Autodesk Inventor part; units mm, degrees
(part 2 of 2)
  spline S369 degree 3 poles (263.9908, 122.8577) (263.1328, 122.8577) (262.3593, 122.3409) (262.031, 121.5482) knots 0 0 0 0 1 1 1 1 projected
  spline S370 degree 3 poles (262.4908, 119.2364) (263.0975, 118.6297) (264.0099, 118.4482) (264.8026, 118.7766) knots 0 0 0 0 1 1 1 1 projected
  spline S371 degree 3 poles (265.4908, 122.2364) (265.093, 122.6342) (264.5534, 122.8577) (263.9908, 122.8577) knots 0 0 0 0 1 1 1 1 projected
  spline S372 degree 3 poles (266.1121, 120.7364) (266.1121, 121.299) (265.8886, 121.8386) (265.4908, 122.2364) knots 0 0 0 0 1 1 1 1 projected
  spline S373 degree 3 poles (264.8026, 118.7766) (265.5953, 119.1049) (266.1121, 119.8784) (266.1121, 120.7364) knots 0 0 0 0 1 1 1 1 projected
  spline S374 degree 3 poles (252.3068, 94.2009) (251.4488, 94.2009) (250.6753, 93.6841) (250.347, 92.8914) knots 0 0 0 0 1 1 1 1 projected
  spline S375 degree 3 poles (250.347, 92.8914) (250.0186, 92.0987) (250.2001, 91.1863) (250.8068, 90.5796) knots 0 0 0 0 1 1 1 1 projected
  spline S376 degree 3 poles (253.8068, 93.5796) (253.409, 93.9774) (252.8694, 94.2009) (252.3068, 94.2009) knots 0 0 0 0 1 1 1 1 projected
  spline S377 degree 3 poles (254.4281, 92.0796) (254.4281, 92.6422) (254.2046, 93.1818) (253.8068, 93.5796) knots 0 0 0 0 1 1 1 1 projected
  spline S378 degree 3 poles (253.1186, 90.1198) (253.9113, 90.4481) (254.4281, 91.2216) (254.4281, 92.0796) knots 0 0 0 0 1 1 1 1 projected
  spline S379 degree 3 poles (250.8068, 90.5796) (251.4135, 89.9729) (252.3259, 89.7914) (253.1186, 90.1198) knots 0 0 0 0 1 1 1 1 projected
  spline S380 degree 3 poles (249.25, 11.25) (249.25, 11.7141) (249.0656, 12.1592) (248.7374, 12.4874) knots 0 0 0 0 1 1 1 1 projected
  spline S381 degree 3 poles (248.1697, 9.6332) (248.8236, 9.9041) (249.25, 10.5422) (249.25, 11.25) knots 0 0 0 0 1 1 1 1 projected
  spline S382 degree 3 poles (257.9446, 32.9698) (258.7373, 33.2981) (259.2541, 34.0716) (259.2541, 34.9296) knots 0 0 0 0 1 1 1 1 projected
  spline S383 degree 3 poles (248.7374, 12.4874) (248.4092, 12.8156) (247.9641, 13) (247.5, 13) knots 0 0 0 0 1 1 1 1 projected
  spline S384 degree 3 poles (246.2626, 10.0126) (246.7631, 9.5121) (247.5158, 9.3623) (248.1697, 9.6332) knots 0 0 0 0 1 1 1 1 projected
  spline S385 degree 3 poles (247.5, 13) (246.7922, 13) (246.1541, 12.5736) (245.8832, 11.9197) knots 0 0 0 0 1 1 1 1 projected
  spline S386 degree 3 poles (245.8832, 107.0581) (245.6123, 106.4042) (245.7621, 105.6515) (246.2626, 105.151) knots 0 0 0 0 1 1 1 1 projected
  spline S387 degree 3 poles (245.8832, 11.9197) (245.6123, 11.2658) (245.7621, 10.5131) (246.2626, 10.0126) knots 0 0 0 0 1 1 1 1 projected
  spline S388 degree 3 poles (255.173, 35.7414) (254.8446, 34.9487) (255.0261, 34.0363) (255.6328, 33.4296) knots 0 0 0 0 1 1 1 1 projected
  line L32 (240.6245, 24.8046) -> (240.6245, 9.8046) projected
  spline S389 degree 3 poles (259.2541, 34.9296) (259.2541, 35.4922) (259.0306, 36.0318) (258.6328, 36.4296) knots 0 0 0 0 1 1 1 1 projected
  line L33 (234.6245, 24.8046) -> (240.6245, 24.8046) projected
  spline S390 degree 3 poles (239.5768, 36.4076) (239.179, 36.8054) (238.6394, 37.0289) (238.0768, 37.0289) knots 0 0 0 0 1 1 1 1 projected
  spline S391 degree 3 poles (240.1981, 34.9076) (240.1981, 35.4702) (239.9746, 36.0098) (239.5768, 36.4076) knots 0 0 0 0 1 1 1 1 projected
  spline S392 degree 3 poles (238.8886, 32.9478) (239.6813, 33.2761) (240.1981, 34.0496) (240.1981, 34.9076) knots 0 0 0 0 1 1 1 1 projected
  spline S393 degree 3 poles (236.5768, 33.4076) (237.1835, 32.8009) (238.0959, 32.6194) (238.8886, 32.9478) knots 0 0 0 0 1 1 1 1 projected
  spline S394 degree 3 poles (236.117, 35.7194) (235.7886, 34.9267) (235.9701, 34.0143) (236.5768, 33.4076) knots 0 0 0 0 1 1 1 1 projected
  spline S395 degree 3 poles (238.0768, 37.0289) (237.2188, 37.0289) (236.4453, 36.5121) (236.117, 35.7194) knots 0 0 0 0 1 1 1 1 projected
  spline S396 degree 3 poles (249.8561, 53.9796) (249.8561, 54.5422) (249.6326, 55.0818) (249.2348, 55.4796) knots 0 0 0 0 1 1 1 1 projected
  spline S397 degree 3 poles (248.5466, 52.0198) (249.3393, 52.3481) (249.8561, 53.1216) (249.8561, 53.9796) knots 0 0 0 0 1 1 1 1 projected
  spline S398 degree 3 poles (249.2348, 55.4796) (248.837, 55.8774) (248.2974, 56.1009) (247.7348, 56.1009) knots 0 0 0 0 1 1 1 1 projected
  spline S399 degree 3 poles (246.2348, 52.4796) (246.8415, 51.8729) (247.7539, 51.6914) (248.5466, 52.0198) knots 0 0 0 0 1 1 1 1 projected
  spline S400 degree 3 poles (247.7348, 56.1009) (246.8768, 56.1009) (246.1033, 55.5841) (245.775, 54.7914) knots 0 0 0 0 1 1 1 1 projected
  spline S401 degree 3 poles (230.5521, 53.9796) (230.5521, 54.5422) (230.3286, 55.0818) (229.9308, 55.4796) knots 0 0 0 0 1 1 1 1 projected
  spline S402 degree 3 poles (229.2426, 52.0198) (230.0353, 52.3481) (230.5521, 53.1216) (230.5521, 53.9796) knots 0 0 0 0 1 1 1 1 projected
  spline S403 degree 3 poles (229.9308, 55.4796) (229.533, 55.8774) (228.9934, 56.1009) (228.4308, 56.1009) knots 0 0 0 0 1 1 1 1 projected
  spline S404 degree 3 poles (245.775, 54.7914) (245.4466, 53.9987) (245.6281, 53.0863) (246.2348, 52.4796) knots 0 0 0 0 1 1 1 1 projected
  spline S405 degree 3 poles (225.1048, 74.5296) (224.707, 74.9274) (224.1674, 75.1509) (223.6048, 75.1509) knots 0 0 0 0 1 1 1 1 projected
  spline S406 degree 3 poles (223.6048, 75.1509) (222.7468, 75.1509) (221.9733, 74.6341) (221.645, 73.8414) knots 0 0 0 0 1 1 1 1 projected
  spline S407 degree 3 poles (225.7261, 73.0296) (225.7261, 73.5922) (225.5026, 74.1318) (225.1048, 74.5296) knots 0 0 0 0 1 1 1 1 projected
  spline S408 degree 3 poles (221.645, 73.8414) (221.3166, 73.0487) (221.4981, 72.1363) (222.1048, 71.5296) knots 0 0 0 0 1 1 1 1 projected
  spline S409 degree 3 poles (222.1048, 71.5296) (222.7115, 70.9229) (223.6239, 70.7414) (224.4166, 71.0698) knots 0 0 0 0 1 1 1 1 projected
  spline S410 degree 3 poles (224.4166, 71.0698) (225.2093, 71.3981) (225.7261, 72.1716) (225.7261, 73.0296) knots 0 0 0 0 1 1 1 1 projected
  spline S411 degree 3 poles (244.1548, 74.5296) (243.757, 74.9274) (243.2174, 75.1509) (242.6548, 75.1509) knots 0 0 0 0 1 1 1 1 projected
  spline S412 degree 3 poles (240.695, 73.8414) (240.3666, 73.0487) (240.5481, 72.1363) (241.1548, 71.5296) knots 0 0 0 0 1 1 1 1 projected
  spline S413 degree 3 poles (244.7761, 73.0296) (244.7761, 73.5922) (244.5526, 74.1318) (244.1548, 74.5296) knots 0 0 0 0 1 1 1 1 projected
  spline S414 degree 3 poles (241.1548, 71.5296) (241.7615, 70.9229) (242.6739, 70.7414) (243.4666, 71.0698) knots 0 0 0 0 1 1 1 1 projected
  spline S415 degree 3 poles (243.4666, 71.0698) (244.2593, 71.3981) (244.7761, 72.1716) (244.7761, 73.0296) knots 0 0 0 0 1 1 1 1 projected
  spline S416 degree 3 poles (242.6548, 75.1509) (241.7968, 75.1509) (241.0233, 74.6341) (240.695, 73.8414) knots 0 0 0 0 1 1 1 1 projected
  spline S417 degree 3 poles (241.6148, 122.2364) (241.217, 122.6342) (240.6774, 122.8577) (240.1148, 122.8577) knots 0 0 0 0 1 1 1 1 projected
  spline S418 degree 3 poles (242.2361, 120.7364) (242.2361, 121.299) (242.0126, 121.8386) (241.6148, 122.2364) knots 0 0 0 0 1 1 1 1 projected
  spline S419 degree 3 poles (240.9266, 118.7766) (241.7193, 119.1049) (242.2361, 119.8784) (242.2361, 120.7364) knots 0 0 0 0 1 1 1 1 projected
  spline S420 degree 3 poles (238.6148, 119.2364) (239.2215, 118.6297) (240.1339, 118.4482) (240.9266, 118.7766) knots 0 0 0 0 1 1 1 1 projected
  spline S421 degree 3 poles (240.1148, 122.8577) (239.2568, 122.8577) (238.4833, 122.3409) (238.155, 121.5482) knots 0 0 0 0 1 1 1 1 projected
  spline S422 degree 3 poles (238.155, 121.5482) (237.8266, 120.7555) (238.0081, 119.8431) (238.6148, 119.2364) knots 0 0 0 0 1 1 1 1 projected
  spline S423 degree 3 poles (235.3781, 92.0796) (235.3781, 92.6422) (235.1546, 93.1818) (234.7568, 93.5796) knots 0 0 0 0 1 1 1 1 projected
  spline S424 degree 3 poles (234.0686, 90.1198) (234.8613, 90.4481) (235.3781, 91.2216) (235.3781, 92.0796) knots 0 0 0 0 1 1 1 1 projected
  spline S425 degree 3 poles (234.7568, 93.5796) (234.359, 93.9774) (233.8194, 94.2009) (233.2568, 94.2009) knots 0 0 0 0 1 1 1 1 projected
  spline S426 degree 3 poles (231.7568, 90.5796) (232.3635, 89.9729) (233.2759, 89.7914) (234.0686, 90.1198) knots 0 0 0 0 1 1 1 1 projected
  spline S427 degree 3 poles (233.2568, 94.2009) (232.3988, 94.2009) (231.6253, 93.6841) (231.297, 92.8914) knots 0 0 0 0 1 1 1 1 projected
  spline S428 degree 3 poles (231.297, 92.8914) (230.9686, 92.0987) (231.1501, 91.1863) (231.7568, 90.5796) knots 0 0 0 0 1 1 1 1 projected
  spline S429 degree 3 poles (216.3281, 92.0796) (216.3281, 92.6422) (216.1046, 93.1818) (215.7068, 93.5796) knots 0 0 0 0 1 1 1 1 projected
  spline S430 degree 3 poles (215.0186, 90.1198) (215.8113, 90.4481) (216.3281, 91.2216) (216.3281, 92.0796) knots 0 0 0 0 1 1 1 1 projected
  spline S431 degree 3 poles (215.7068, 93.5796) (215.309, 93.9774) (214.7694, 94.2009) (214.2068, 94.2009) knots 0 0 0 0 1 1 1 1 projected
  spline S432 degree 3 poles (212.7068, 90.5796) (213.3135, 89.9729) (214.2259, 89.7914) (215.0186, 90.1198) knots 0 0 0 0 1 1 1 1 projected
  spline S433 degree 3 poles (212.247, 92.8914) (211.9186, 92.0987) (212.1001, 91.1863) (212.7068, 90.5796) knots 0 0 0 0 1 1 1 1 projected
  spline S434 degree 3 poles (214.2068, 94.2009) (213.3488, 94.2009) (212.5753, 93.6841) (212.247, 92.8914) knots 0 0 0 0 1 1 1 1 projected
  spline S435 degree 3 poles (217.0506, 118.7766) (217.8433, 119.1049) (218.3601, 119.8784) (218.3601, 120.7364) knots 0 0 0 0 1 1 1 1 projected
  spline S436 degree 3 poles (218.3601, 120.7364) (218.3601, 121.299) (218.1366, 121.8386) (217.7388, 122.2364) knots 0 0 0 0 1 1 1 1 projected
  spline S437 degree 3 poles (214.7388, 119.2364) (215.3455, 118.6297) (216.2579, 118.4482) (217.0506, 118.7766) knots 0 0 0 0 1 1 1 1 projected
  spline S438 degree 3 poles (217.7388, 122.2364) (217.341, 122.6342) (216.8014, 122.8577) (216.2388, 122.8577) knots 0 0 0 0 1 1 1 1 projected
  spline S439 degree 3 poles (216.2388, 122.8577) (215.3808, 122.8577) (214.6073, 122.3409) (214.279, 121.5482) knots 0 0 0 0 1 1 1 1 projected
  spline S440 degree 3 poles (214.279, 121.5482) (213.9506, 120.7555) (214.1321, 119.8431) (214.7388, 119.2364) knots 0 0 0 0 1 1 1 1 projected
  spline S441 degree 3 poles (221.1581, 34.9276) (221.1581, 36.0992) (220.2084, 37.0489) (219.0368, 37.0489) knots 0 0 0 0 1 1 1 1 projected
  spline S442 degree 3 poles (219.8486, 32.9678) (220.6413, 33.2961) (221.1581, 34.0696) (221.1581, 34.9276) knots 0 0 0 0 1 1 1 1 projected
  spline S443 degree 3 poles (217.5368, 33.4276) (218.1435, 32.8209) (219.0559, 32.6394) (219.8486, 32.9678) knots 0 0 0 0 1 1 1 1 projected
  spline S444 degree 3 poles (217.077, 35.7394) (216.7486, 34.9467) (216.9301, 34.0343) (217.5368, 33.4276) knots 0 0 0 0 1 1 1 1 projected
  spline S445 degree 3 poles (219.0368, 37.0489) (218.1788, 37.0489) (217.4053, 36.5321) (217.077, 35.7394) knots 0 0 0 0 1 1 1 1 projected
  spline S446 degree 3 poles (228.4308, 56.1009) (227.5728, 56.1009) (226.7993, 55.5841) (226.471, 54.7914) knots 0 0 0 0 1 1 1 1 projected
  spline S447 degree 3 poles (226.471, 54.7914) (226.1426, 53.9987) (226.3241, 53.0863) (226.9308, 52.4796) knots 0 0 0 0 1 1 1 1 projected
  spline S448 degree 3 poles (226.9308, 52.4796) (227.5375, 51.8729) (228.4499, 51.6914) (229.2426, 52.0198) knots 0 0 0 0 1 1 1 1 projected
  spline S449 degree 3 poles (211.5021, 53.9796) (211.5021, 54.5422) (211.2786, 55.0818) (210.8808, 55.4796) knots 0 0 0 0 1 1 1 1 projected
  spline S450 degree 3 poles (210.1926, 52.0198) (210.9853, 52.3481) (211.5021, 53.1216) (211.5021, 53.9796) knots 0 0 0 0 1 1 1 1 projected
  spline S451 degree 3 poles (209.3808, 56.1009) (208.5228, 56.1009) (207.7493, 55.5841) (207.421, 54.7914) knots 0 0 0 0 1 1 1 1 projected
  spline S452 degree 3 poles (207.8808, 52.4796) (208.4875, 51.8729) (209.3999, 51.6914) (210.1926, 52.0198) knots 0 0 0 0 1 1 1 1 projected
  spline S453 degree 3 poles (207.421, 54.7914) (207.0926, 53.9987) (207.2741, 53.0863) (207.8808, 52.4796) knots 0 0 0 0 1 1 1 1 projected
  spline S454 degree 3 poles (210.8808, 55.4796) (210.483, 55.8774) (209.9434, 56.1009) (209.3808, 56.1009) knots 0 0 0 0 1 1 1 1 projected
  line L34 (298.1708, 72.3776) -> (298.1708, 78.3776) projected
  line L35 (298.1708, 78.3776) -> (313.1708, 78.3776) projected
  line L36 (313.1708, 78.3776) -> (313.1708, 72.3776) projected
  line L37 (298.1708, 54.3776) -> (313.1708, 54.3776) projected
  line L38 (298.1708, 48.3776) -> (298.1708, 54.3776) projected
  line L39 (313.1708, 48.3776) -> (298.1708, 48.3776) projected
  line L40 (313.1708, 54.3776) -> (313.1708, 48.3776) projected
  line L41 (301.9468, 43.9296) -> (307.9468, 43.9296) projected
  spline S455 degree 3 poles (292.9468, 37.0509) (292.0888, 37.0509) (291.3153, 36.5341) (290.987, 35.7414) knots 0 0 0 0 1 1 1 1 projected
  spline S456 degree 3 poles (293.7586, 32.9698) (294.5513, 33.2981) (295.0681, 34.0716) (295.0681, 34.9296) knots 0 0 0 0 1 1 1 1 projected
  line L42 (277.9468, 43.9296) -> (283.9468, 43.9296) projected
  spline S457 degree 3 poles (291.4468, 33.4296) (292.0535, 32.8229) (292.9659, 32.6414) (293.7586, 32.9698) knots 0 0 0 0 1 1 1 1 projected
  line L43 (301.9468, 28.9296) -> (301.9468, 43.9296) projected
  line L44 (307.9468, 28.9296) -> (301.9468, 28.9296) projected
  line L45 (307.9468, 43.9296) -> (307.9468, 28.9296) projected
  line L46 (277.9468, 28.9296) -> (277.9468, 43.9296) projected
  line L47 (283.9468, 28.9296) -> (277.9468, 28.9296) projected
  spline S458 degree 3 poles (258.6328, 36.4296) (258.235, 36.8274) (257.6954, 37.0509) (257.1328, 37.0509) knots 0 0 0 0 1 1 1 1 projected
  spline S459 degree 3 poles (257.1328, 37.0509) (256.2748, 37.0509) (255.5013, 36.5341) (255.173, 35.7414) knots 0 0 0 0 1 1 1 1 projected
  spline S460 degree 3 poles (248.1697, 104.7716) (248.8236, 105.0425) (249.25, 105.6806) (249.25, 106.3884) knots 0 0 0 0 1 1 1 1 projected
  spline S461 degree 3 poles (249.25, 106.3884) (249.25, 106.8525) (249.0656, 107.2976) (248.7374, 107.6258) knots 0 0 0 0 1 1 1 1 projected
  spline S462 degree 3 poles (246.2626, 105.151) (246.7631, 104.6505) (247.5158, 104.5007) (248.1697, 104.7716) knots 0 0 0 0 1 1 1 1 projected
  spline S463 degree 3 poles (266.603, 16.6914) (266.2746, 15.8987) (266.4561, 14.9863) (267.0628, 14.3796) knots 0 0 0 0 1 1 1 1 projected
  spline S464 degree 3 poles (248.7374, 107.6258) (248.4092, 107.954) (247.9641, 108.1384) (247.5, 108.1384) knots 0 0 0 0 1 1 1 1 projected
  spline S465 degree 3 poles (247.5, 108.1384) (246.7922, 108.1384) (246.1541, 107.712) (245.8832, 107.0581) knots 0 0 0 0 1 1 1 1 projected
  line L48 (240.6245, 9.8046) -> (234.6245, 9.8046) projected
  line L49 (234.6245, 9.8046) -> (234.6245, 24.8046) projected
  line L50 (467.2088, 40.476) -> (452.2088, 40.476) projected
  line L51 (467.2088, 34.476) -> (467.2088, 40.476) projected
  line L52 (452.2088, 34.476) -> (467.2088, 34.476) projected
  line L53 (22.5, 6.25) -> (472.5, 6.25) projected
  line L54 (22.5, 131.25) -> (472.5, 131.25) projected
  line L55 (22.5, 131.25) -> (22.5, 6.25) projected
  spline S466 degree 3 poles (25.8832, 44.9197) (25.6123, 44.2658) (25.7621, 43.5131) (26.2626, 43.0126) knots 0 0 0 0 1 1 1 1 projected
  spline S467 degree 3 poles (27.5, 46) (26.7922, 46) (26.1541, 45.5736) (25.8832, 44.9197) knots 0 0 0 0 1 1 1 1 projected
  spline S468 degree 3 poles (319.4023, 126.7719) (318.4647, 127.7096) (317.1929, 128.2364) (315.8668, 128.2364) knots 0 0 0 0 1 1 1 1 projected
  spline S469 degree 3 poles (320.8668, 123.2364) (320.8668, 124.5625) (320.34, 125.8343) (319.4023, 126.7719) knots 0 0 0 0 1 1 1 1 projected
  spline S470 degree 3 poles (317.7802, 118.617) (319.6486, 119.3909) (320.8668, 121.2141) (320.8668, 123.2364) knots 0 0 0 0 1 1 1 1 projected
  spline S471 degree 3 poles (312.3313, 119.7009) (313.7613, 118.2709) (315.9118, 117.8431) (317.7802, 118.617) knots 0 0 0 0 1 1 1 1 projected
  spline S472 degree 3 poles (311.2474, 125.1498) (310.4735, 123.2814) (310.9013, 121.1309) (312.3313, 119.7009) knots 0 0 0 0 1 1 1 1 projected
  spline S473 degree 3 poles (315.8668, 128.2364) (313.8445, 128.2364) (312.0213, 127.0182) (311.2474, 125.1498) knots 0 0 0 0 1 1 1 1 projected
  spline S474 degree 3 poles (310.9568, 93.5796) (310.559, 93.9774) (310.0194, 94.2009) (309.4568, 94.2009) knots 0 0 0 0 1 1 1 1 projected
  spline S475 degree 3 poles (311.5781, 92.0796) (311.5781, 92.6422) (311.3546, 93.1818) (310.9568, 93.5796) knots 0 0 0 0 1 1 1 1 projected
  spline S476 degree 3 poles (309.4568, 89.9583) (310.6284, 89.9583) (311.5781, 90.908) (311.5781, 92.0796) knots 0 0 0 0 1 1 1 1 projected
  spline S477 degree 3 poles (307.3355, 92.0796) (307.3355, 90.908) (308.2852, 89.9583) (309.4568, 89.9583) knots 0 0 0 0 1 1 1 1 projected
  spline S478 degree 3 poles (309.4568, 94.2009) (308.2852, 94.2009) (307.3355, 93.2512) (307.3355, 92.0796) knots 0 0 0 0 1 1 1 1 projected
  spline S479 degree 3 poles (289.3668, 122.2364) (288.969, 122.6342) (288.4294, 122.8577) (287.8668, 122.8577) knots 0 0 0 0 1 1 1 1 projected
  spline S480 degree 3 poles (289.9881, 120.7364) (289.9881, 121.299) (289.7646, 121.8386) (289.3668, 122.2364) knots 0 0 0 0 1 1 1 1 projected
  spline S481 degree 3 poles (287.8668, 118.6151) (289.0384, 118.6151) (289.9881, 119.5648) (289.9881, 120.7364) knots 0 0 0 0 1 1 1 1 projected
  spline S482 degree 3 poles (285.7455, 120.7364) (285.7455, 119.5648) (286.6952, 118.6151) (287.8668, 118.6151) knots 0 0 0 0 1 1 1 1 projected
  spline S483 degree 3 poles (287.8668, 122.8577) (286.6952, 122.8577) (285.7455, 121.908) (285.7455, 120.7364) knots 0 0 0 0 1 1 1 1 projected
  spline S484 degree 3 poles (272.8568, 93.5796) (272.459, 93.9774) (271.9194, 94.2009) (271.3568, 94.2009) knots 0 0 0 0 1 1 1 1 projected
  spline S485 degree 3 poles (273.4781, 92.0796) (273.4781, 92.6422) (273.2546, 93.1818) (272.8568, 93.5796) knots 0 0 0 0 1 1 1 1 projected
  spline S486 degree 3 poles (272.1686, 90.1198) (272.9613, 90.4481) (273.4781, 91.2216) (273.4781, 92.0796) knots 0 0 0 0 1 1 1 1 projected
  spline S487 degree 3 poles (269.8568, 90.5796) (270.4635, 89.9729) (271.3759, 89.7914) (272.1686, 90.1198) knots 0 0 0 0 1 1 1 1 projected
  spline S488 degree 3 poles (269.397, 92.8914) (269.0686, 92.0987) (269.2501, 91.1863) (269.8568, 90.5796) knots 0 0 0 0 1 1 1 1 projected
  spline S489 degree 3 poles (271.3568, 94.2009) (270.4988, 94.2009) (269.7253, 93.6841) (269.397, 92.8914) knots 0 0 0 0 1 1 1 1 projected
  spline S490 degree 3 poles (288.447, 92.8914) (288.1186, 92.0987) (288.3001, 91.1863) (288.9068, 90.5796) knots 0 0 0 0 1 1 1 1 projected
  spline S491 degree 3 poles (290.4068, 94.2009) (289.5488, 94.2009) (288.7753, 93.6841) (288.447, 92.8914) knots 0 0 0 0 1 1 1 1 projected
  spline S492 degree 3 poles (288.9068, 90.5796) (289.5135, 89.9729) (290.4259, 89.7914) (291.2186, 90.1198) knots 0 0 0 0 1 1 1 1 projected
  spline S493 degree 3 poles (292.5281, 92.0796) (292.5281, 92.6422) (292.3046, 93.1818) (291.9068, 93.5796) knots 0 0 0 0 1 1 1 1 projected
  spline S494 degree 3 poles (291.2186, 90.1198) (292.0113, 90.4481) (292.5281, 91.2216) (292.5281, 92.0796) knots 0 0 0 0 1 1 1 1 projected
  spline S495 degree 3 poles (291.9068, 93.5796) (291.509, 93.9774) (290.9694, 94.2009) (290.4068, 94.2009) knots 0 0 0 0 1 1 1 1 projected
  spline S496 degree 3 poles (357.88, 36.4804) (357.4822, 36.8782) (356.9426, 37.1017) (356.38, 37.1017) knots 0 0 0 0 1 1 1 1 projected
  spline S497 degree 3 poles (358.5013, 34.9804) (358.5013, 35.543) (358.2778, 36.0826) (357.88, 36.4804) knots 0 0 0 0 1 1 1 1 projected
  spline S498 degree 3 poles (357.1918, 33.0206) (357.9845, 33.3489) (358.5013, 34.1224) (358.5013, 34.9804) knots 0 0 0 0 1 1 1 1 projected
  spline S499 degree 3 poles (354.88, 33.4804) (355.4867, 32.8737) (356.3991, 32.6922) (357.1918, 33.0206) knots 0 0 0 0 1 1 1 1 projected
  spline S500 degree 3 poles (356.38, 37.1017) (355.522, 37.1017) (354.7485, 36.5849) (354.4202, 35.7922) knots 0 0 0 0 1 1 1 1 projected
  spline S501 degree 3 poles (354.88, 52.5304) (355.4867, 51.9237) (356.3991, 51.7422) (357.1918, 52.0706) knots 0 0 0 0 1 1 1 1 projected
  spline S502 degree 3 poles (354.4202, 54.8422) (354.0918, 54.0495) (354.2733, 53.1371) (354.88, 52.5304) knots 0 0 0 0 1 1 1 1 projected
  spline S503 degree 3 poles (356.38, 56.1517) (355.522, 56.1517) (354.7485, 55.6349) (354.4202, 54.8422) knots 0 0 0 0 1 1 1 1 projected
  spline S504 degree 3 poles (357.88, 55.5304) (357.4822, 55.9282) (356.9426, 56.1517) (356.38, 56.1517) knots 0 0 0 0 1 1 1 1 projected
  spline S505 degree 3 poles (358.5013, 54.0304) (358.5013, 54.593) (358.2778, 55.1326) (357.88, 55.5304) knots 0 0 0 0 1 1 1 1 projected
  spline S506 degree 3 poles (357.1918, 52.0706) (357.9845, 52.3989) (358.5013, 53.1724) (358.5013, 54.0304) knots 0 0 0 0 1 1 1 1 projected
  spline S507 degree 3 poles (354.4202, 35.7922) (354.0918, 34.9995) (354.2733, 34.0871) (354.88, 33.4804) knots 0 0 0 0 1 1 1 1 projected
  spline S508 degree 3 poles (343.558, 93.6444) (343.1602, 94.0422) (342.6206, 94.2657) (342.058, 94.2657) knots 0 0 0 0 1 1 1 1 projected
  spline S509 degree 3 poles (344.1793, 92.1444) (344.1793, 92.707) (343.9558, 93.2466) (343.558, 93.6444) knots 0 0 0 0 1 1 1 1 projected
  spline S510 degree 3 poles (342.8698, 90.1846) (343.6625, 90.5129) (344.1793, 91.2864) (344.1793, 92.1444) knots 0 0 0 0 1 1 1 1 projected
  spline S511 degree 3 poles (340.558, 90.6444) (341.1647, 90.0377) (342.0771, 89.8562) (342.8698, 90.1846) knots 0 0 0 0 1 1 1 1 projected
  spline S512 degree 3 poles (340.0982, 92.9562) (339.7698, 92.1635) (339.9513, 91.2511) (340.558, 90.6444) knots 0 0 0 0 1 1 1 1 projected
  spline S513 degree 3 poles (342.058, 94.2657) (341.2, 94.2657) (340.4265, 93.7489) (340.0982, 92.9562) knots 0 0 0 0 1 1 1 1 projected
  spline S514 degree 3 poles (369.154, 90.6444) (369.7607, 90.0377) (370.6731, 89.8562) (371.4658, 90.1846) knots 0 0 0 0 1 1 1 1 projected
  spline S515 degree 3 poles (368.6942, 92.9562) (368.3658, 92.1635) (368.5473, 91.2511) (369.154, 90.6444) knots 0 0 0 0 1 1 1 1 projected
  spline S516 degree 3 poles (371.4658, 90.1846) (372.2585, 90.5129) (372.7753, 91.2864) (372.7753, 92.1444) knots 0 0 0 0 1 1 1 1 projected
  spline S517 degree 3 poles (372.7753, 92.1444) (372.7753, 92.707) (372.5518, 93.2466) (372.154, 93.6444) knots 0 0 0 0 1 1 1 1 projected
  spline S518 degree 3 poles (372.154, 93.6444) (371.7562, 94.0422) (371.2166, 94.2657) (370.654, 94.2657) knots 0 0 0 0 1 1 1 1 projected
  spline S519 degree 3 poles (370.654, 94.2657) (369.796, 94.2657) (369.0225, 93.7489) (368.6942, 92.9562) knots 0 0 0 0 1 1 1 1 projected
  spline S520 degree 3 poles (358.7374, 12.4874) (358.4092, 12.8156) (357.9641, 13) (357.5, 13) knots 0 0 0 0 1 1 1 1 projected
  spline S521 degree 3 poles (359.25, 11.25) (359.25, 11.7141) (359.0656, 12.1592) (358.7374, 12.4874) knots 0 0 0 0 1 1 1 1 projected
  spline S522 degree 3 poles (358.1697, 9.6332) (358.8236, 9.9041) (359.25, 10.5422) (359.25, 11.25) knots 0 0 0 0 1 1 1 1 projected
  spline S523 degree 3 poles (356.2626, 10.0126) (356.7631, 9.5121) (357.5158, 9.3623) (358.1697, 9.6332) knots 0 0 0 0 1 1 1 1 projected
  spline S524 degree 3 poles (355.8832, 11.9197) (355.6123, 11.2658) (355.7621, 10.5131) (356.2626, 10.0126) knots 0 0 0 0 1 1 1 1 projected
  spline S525 degree 3 poles (357.5, 13) (356.7922, 13) (356.1541, 12.5736) (355.8832, 11.9197) knots 0 0 0 0 1 1 1 1 projected
  spline S526 degree 3 poles (373.3087, 34.9804) (373.3087, 33.8088) (374.2584, 32.8591) (375.43, 32.8591) knots 0 0 0 0 1 1 1 1 projected
  spline S527 degree 3 poles (376.93, 36.4804) (376.5322, 36.8782) (375.9926, 37.1017) (375.43, 37.1017) knots 0 0 0 0 1 1 1 1 projected
  spline S528 degree 3 poles (375.43, 32.8591) (376.6016, 32.8591) (377.5513, 33.8088) (377.5513, 34.9804) knots 0 0 0 0 1 1 1 1 projected
  spline S529 degree 3 poles (377.5513, 34.9804) (377.5513, 35.543) (377.3278, 36.0826) (376.93, 36.4804) knots 0 0 0 0 1 1 1 1 projected
  spline S530 degree 3 poles (375.43, 37.1017) (374.2584, 37.1017) (373.3087, 36.152) (373.3087, 34.9804) knots 0 0 0 0 1 1 1 1 projected
  spline S531 degree 3 poles (405.5588, 93.678) (405.161, 94.0758) (404.6214, 94.2993) (404.0588, 94.2993) knots 0 0 0 0 1 1 1 1 projected
  spline S532 degree 3 poles (406.1801, 92.178) (406.1801, 92.7406) (405.9566, 93.2802) (405.5588, 93.678) knots 0 0 0 0 1 1 1 1 projected
  spline S533 degree 3 poles (404.8706, 90.2182) (405.6633, 90.5465) (406.1801, 91.32) (406.1801, 92.178) knots 0 0 0 0 1 1 1 1 projected
  spline S534 degree 3 poles (402.5588, 90.678) (403.1655, 90.0713) (404.0779, 89.8898) (404.8706, 90.2182) knots 0 0 0 0 1 1 1 1 projected
  spline S535 degree 3 poles (402.099, 92.9898) (401.7706, 92.1971) (401.9521, 91.2847) (402.5588, 90.678) knots 0 0 0 0 1 1 1 1 projected
  spline S536 degree 3 poles (404.0588, 94.2993) (403.2008, 94.2993) (402.4273, 93.7825) (402.099, 92.9898) knots 0 0 0 0 1 1 1 1 projected
  spline S537 degree 3 poles (424.6088, 55.578) (424.211, 55.9758) (423.6714, 56.1993) (423.1088, 56.1993) knots 0 0 0 0 1 1 1 1 projected
  spline S538 degree 3 poles (425.2301, 54.078) (425.2301, 54.6406) (425.0066, 55.1802) (424.6088, 55.578) knots 0 0 0 0 1 1 1 1 projected
  spline S539 degree 3 poles (423.9206, 52.1182) (424.7133, 52.4465) (425.2301, 53.22) (425.2301, 54.078) knots 0 0 0 0 1 1 1 1 projected
  spline S540 degree 3 poles (421.6088, 52.578) (422.2155, 51.9713) (423.1279, 51.7898) (423.9206, 52.1182) knots 0 0 0 0 1 1 1 1 projected
  spline S541 degree 3 poles (421.149, 54.8898) (420.8206, 54.0971) (421.0021, 53.1847) (421.6088, 52.578) knots 0 0 0 0 1 1 1 1 projected
  spline S542 degree 3 poles (423.1088, 56.1993) (422.2508, 56.1993) (421.4773, 55.6825) (421.149, 54.8898) knots 0 0 0 0 1 1 1 1 projected
  spline S543 degree 3 poles (402.5588, 52.578) (403.1655, 51.9713) (404.0779, 51.7898) (404.8706, 52.1182) knots 0 0 0 0 1 1 1 1 projected
  spline S544 degree 3 poles (404.8706, 52.1182) (405.6633, 52.4465) (406.1801, 53.22) (406.1801, 54.078) knots 0 0 0 0 1 1 1 1 projected
  spline S545 degree 3 poles (402.099, 54.8898) (401.7706, 54.0971) (401.9521, 53.1847) (402.5588, 52.578) knots 0 0 0 0 1 1 1 1 projected
  spline S546 degree 3 poles (406.1801, 54.078) (406.1801, 54.6406) (405.9566, 55.1802) (405.5588, 55.578) knots 0 0 0 0 1 1 1 1 projected
  spline S547 degree 3 poles (405.5588, 55.578) (405.161, 55.9758) (404.6214, 56.1993) (404.0588, 56.1993) knots 0 0 0 0 1 1 1 1 projected
  spline S548 degree 3 poles (404.0588, 56.1993) (403.2008, 56.1993) (402.4273, 55.6825) (402.099, 54.8898) knots 0 0 0 0 1 1 1 1 projected
  spline S549 degree 3 poles (421.6088, 71.628) (422.2155, 71.0213) (423.1279, 70.8398) (423.9206, 71.1682) knots 0 0 0 0 1 1 1 1 projected
  spline S550 degree 3 poles (402.5588, 71.628) (403.1655, 71.0213) (404.0779, 70.8398) (404.8706, 71.1682) knots 0 0 0 0 1 1 1 1 projected
  spline S551 degree 3 poles (404.8706, 71.1682) (405.6633, 71.4965) (406.1801, 72.27) (406.1801, 73.128) knots 0 0 0 0 1 1 1 1 projected
  spline S552 degree 3 poles (402.099, 73.9398) (401.7706, 73.1471) (401.9521, 72.2347) (402.5588, 71.628) knots 0 0 0 0 1 1 1 1 projected
  spline S553 degree 3 poles (406.1801, 73.128) (406.1801, 73.6906) (405.9566, 74.2302) (405.5588, 74.628) knots 0 0 0 0 1 1 1 1 projected
  spline S554 degree 3 poles (404.0588, 75.2493) (403.2008, 75.2493) (402.4273, 74.7325) (402.099, 73.9398) knots 0 0 0 0 1 1 1 1 projected
  spline S555 degree 3 poles (405.5588, 74.628) (405.161, 75.0258) (404.6214, 75.2493) (404.0588, 75.2493) knots 0 0 0 0 1 1 1 1 projected
  spline S556 degree 3 poles (423.9206, 71.1682) (424.7133, 71.4965) (425.2301, 72.27) (425.2301, 73.128) knots 0 0 0 0 1 1 1 1 projected
  spline S557 degree 3 poles (421.149, 73.9398) (420.8206, 73.1471) (421.0021, 72.2347) (421.6088, 71.628) knots 0 0 0 0 1 1 1 1 projected
  spline S558 degree 3 poles (423.1088, 75.2493) (422.2508, 75.2493) (421.4773, 74.7325) (421.149, 73.9398) knots 0 0 0 0 1 1 1 1 projected
  spline S559 degree 3 poles (424.6088, 74.628) (424.211, 75.0258) (423.6714, 75.2493) (423.1088, 75.2493) knots 0 0 0 0 1 1 1 1 projected
  spline S560 degree 3 poles (425.2301, 73.128) (425.2301, 73.6906) (425.0066, 74.2302) (424.6088, 74.628) knots 0 0 0 0 1 1 1 1 projected
  spline S561 degree 3 poles (405.5588, 36.528) (405.161, 36.9258) (404.6214, 37.1493) (404.0588, 37.1493) knots 0 0 0 0 1 1 1 1 projected
  spline S562 degree 3 poles (406.1801, 35.028) (406.1801, 35.5906) (405.9566, 36.1302) (405.5588, 36.528) knots 0 0 0 0 1 1 1 1 projected
  spline S563 degree 3 poles (404.8706, 33.0682) (405.6633, 33.3965) (406.1801, 34.17) (406.1801, 35.028) knots 0 0 0 0 1 1 1 1 projected
  spline S564 degree 3 poles (404.0588, 37.1493) (403.2008, 37.1493) (402.4273, 36.6325) (402.099, 35.8398) knots 0 0 0 0 1 1 1 1 projected
  spline S565 degree 3 poles (402.099, 35.8398) (401.7706, 35.0471) (401.9521, 34.1347) (402.5588, 33.528) knots 0 0 0 0 1 1 1 1 projected
  spline S566 degree 3 poles (402.5588, 33.528) (403.1655, 32.9213) (404.0779, 32.7398) (404.8706, 33.0682) knots 0 0 0 0 1 1 1 1 projected
  spline S567 degree 3 poles (424.6088, 36.528) (424.211, 36.9258) (423.6714, 37.1493) (423.1088, 37.1493) knots 0 0 0 0 1 1 1 1 projected
  spline S568 degree 3 poles (423.1088, 37.1493) (422.2508, 37.1493) (421.4773, 36.6325) (421.149, 35.8398) knots 0 0 0 0 1 1 1 1 projected
  spline S569 degree 3 poles (425.2301, 35.028) (425.2301, 35.5906) (425.0066, 36.1302) (424.6088, 36.528) knots 0 0 0 0 1 1 1 1 projected
  spline S570 degree 3 poles (421.149, 35.8398) (420.8206, 35.0471) (421.0021, 34.1347) (421.6088, 33.528) knots 0 0 0 0 1 1 1 1 projected
  spline S571 degree 3 poles (423.9206, 33.0682) (424.7133, 33.3965) (425.2301, 34.17) (425.2301, 35.028) knots 0 0 0 0 1 1 1 1 projected
  spline S572 degree 3 poles (421.6088, 33.528) (422.2155, 32.9213) (423.1279, 32.7398) (423.9206, 33.0682) knots 0 0 0 0 1 1 1 1 projected
  spline S573 degree 3 poles (413.7108, 18.0993) (412.8528, 18.0993) (412.0793, 17.5825) (411.751, 16.7898) knots 0 0 0 0 1 1 1 1 projected
  spline S574 degree 3 poles (415.8321, 15.978) (415.8321, 16.5406) (415.6086, 17.0802) (415.2108, 17.478) knots 0 0 0 0 1 1 1 1 projected
  spline S575 degree 3 poles (414.5226, 14.0182) (415.3153, 14.3465) (415.8321, 15.12) (415.8321, 15.978) knots 0 0 0 0 1 1 1 1 projected
  spline S576 degree 3 poles (411.751, 16.7898) (411.4226, 15.9971) (411.6041, 15.0847) (412.2108, 14.478) knots 0 0 0 0 1 1 1 1 projected
  spline S577 degree 3 poles (412.2108, 14.478) (412.8175, 13.8713) (413.7299, 13.6898) (414.5226, 14.0182) knots 0 0 0 0 1 1 1 1 projected
  spline S578 degree 3 poles (415.2108, 17.478) (414.813, 17.8758) (414.2734, 18.0993) (413.7108, 18.0993) knots 0 0 0 0 1 1 1 1 projected
  spline S579 degree 3 poles (462.7088, 93.678) (462.311, 94.0758) (461.7714, 94.2993) (461.2088, 94.2993) knots 0 0 0 0 1 1 1 1 projected
  spline S580 degree 3 poles (463.3301, 92.178) (463.3301, 92.7406) (463.1066, 93.2802) (462.7088, 93.678) knots 0 0 0 0 1 1 1 1 projected
  spline S581 degree 3 poles (462.0206, 90.2182) (462.8133, 90.5465) (463.3301, 91.32) (463.3301, 92.178) knots 0 0 0 0 1 1 1 1 projected
  spline S582 degree 3 poles (459.7088, 90.678) (460.3155, 90.0713) (461.2279, 89.8898) (462.0206, 90.2182) knots 0 0 0 0 1 1 1 1 projected
  spline S583 degree 3 poles (459.249, 92.9898) (458.9206, 92.1971) (459.1021, 91.2847) (459.7088, 90.678) knots 0 0 0 0 1 1 1 1 projected
  spline S584 degree 3 poles (461.2088, 94.2993) (460.3508, 94.2993) (459.5773, 93.7825) (459.249, 92.9898) knots 0 0 0 0 1 1 1 1 projected
  spline S585 degree 3 poles (440.6588, 90.678) (441.2655, 90.0713) (442.1779, 89.8898) (442.9706, 90.2182) knots 0 0 0 0 1 1 1 1 projected
  spline S586 degree 3 poles (442.9706, 90.2182) (443.7633, 90.5465) (444.2801, 91.32) (444.2801, 92.178) knots 0 0 0 0 1 1 1 1 projected
  spline S587 degree 3 poles (440.199, 92.9898) (439.8706, 92.1971) (440.0521, 91.2847) (440.6588, 90.678) knots 0 0 0 0 1 1 1 1 projected
  spline S588 degree 3 poles (443.6588, 93.678) (443.261, 94.0758) (442.7214, 94.2993) (442.1588, 94.2993) knots 0 0 0 0 1 1 1 1 projected
  spline S589 degree 3 poles (442.1588, 94.2993) (441.3008, 94.2993) (440.5273, 93.7825) (440.199, 92.9898) knots 0 0 0 0 1 1 1 1 projected
  spline S590 degree 3 poles (423.9206, 90.2182) (424.7133, 90.5465) (425.2301, 91.32) (425.2301, 92.178) knots 0 0 0 0 1 1 1 1 projected
  spline S591 degree 3 poles (421.6088, 90.678) (422.2155, 90.0713) (423.1279, 89.8898) (423.9206, 90.2182) knots 0 0 0 0 1 1 1 1 projected
  spline S592 degree 3 poles (425.2301, 92.178) (425.2301, 92.7406) (425.0066, 93.2802) (424.6088, 93.678) knots 0 0 0 0 1 1 1 1 projected
  spline S593 degree 3 poles (424.6088, 93.678) (424.211, 94.0758) (423.6714, 94.2993) (423.1088, 94.2993) knots 0 0 0 0 1 1 1 1 projected
  spline S594 degree 3 poles (421.149, 92.9898) (420.8206, 92.1971) (421.0021, 91.2847) (421.6088, 90.678) knots 0 0 0 0 1 1 1 1 projected
  spline S595 degree 3 poles (423.1088, 94.2993) (422.2508, 94.2993) (421.4773, 93.7825) (421.149, 92.9898) knots 0 0 0 0 1 1 1 1 projected
  spline S596 degree 3 poles (444.2801, 92.178) (444.2801, 92.7406) (444.0566, 93.2802) (443.6588, 93.678) knots 0 0 0 0 1 1 1 1 projected
  spline S597 degree 3 poles (443.6588, 74.628) (443.261, 75.0258) (442.7214, 75.2493) (442.1588, 75.2493) knots 0 0 0 0 1 1 1 1 projected
  spline S598 degree 3 poles (444.2801, 73.128) (444.2801, 73.6906) (444.0566, 74.2302) (443.6588, 74.628) knots 0 0 0 0 1 1 1 1 projected
  spline S599 degree 3 poles (442.9706, 71.1682) (443.7633, 71.4965) (444.2801, 72.27) (444.2801, 73.128) knots 0 0 0 0 1 1 1 1 projected
  spline S600 degree 3 poles (442.1588, 75.2493) (441.3008, 75.2493) (440.5273, 74.7325) (440.199, 73.9398) knots 0 0 0 0 1 1 1 1 projected
  spline S601 degree 3 poles (440.199, 73.9398) (439.8706, 73.1471) (440.0521, 72.2347) (440.6588, 71.628) knots 0 0 0 0 1 1 1 1 projected
  spline S602 degree 3 poles (440.6588, 71.628) (441.2655, 71.0213) (442.1779, 70.8398) (442.9706, 71.1682) knots 0 0 0 0 1 1 1 1 projected
  spline S603 degree 3 poles (459.249, 73.9398) (458.9206, 73.1471) (459.1021, 72.2347) (459.7088, 71.628) knots 0 0 0 0 1 1 1 1 projected
  spline S604 degree 3 poles (461.2088, 75.2493) (460.3508, 75.2493) (459.5773, 74.7325) (459.249, 73.9398) knots 0 0 0 0 1 1 1 1 projected
  spline S605 degree 3 poles (462.7088, 74.628) (462.311, 75.0258) (461.7714, 75.2493) (461.2088, 75.2493) knots 0 0 0 0 1 1 1 1 projected
  spline S606 degree 3 poles (463.3301, 73.128) (463.3301, 73.6906) (463.1066, 74.2302) (462.7088, 74.628) knots 0 0 0 0 1 1 1 1 projected
  spline S607 degree 3 poles (459.7088, 71.628) (460.3155, 71.0213) (461.2279, 70.8398) (462.0206, 71.1682) knots 0 0 0 0 1 1 1 1 projected
  spline S608 degree 3 poles (462.0206, 71.1682) (462.8133, 71.4965) (463.3301, 72.27) (463.3301, 73.128) knots 0 0 0 0 1 1 1 1 projected
  spline S609 degree 3 poles (443.6588, 55.578) (443.261, 55.9758) (442.7214, 56.1993) (442.1588, 56.1993) knots 0 0 0 0 1 1 1 1 projected
  spline S610 degree 3 poles (442.1588, 56.1993) (441.3008, 56.1993) (440.5273, 55.6825) (440.199, 54.8898) knots 0 0 0 0 1 1 1 1 projected
  spline S611 degree 3 poles (444.2801, 54.078) (444.2801, 54.6406) (444.0566, 55.1802) (443.6588, 55.578) knots 0 0 0 0 1 1 1 1 projected
  spline S612 degree 3 poles (440.199, 54.8898) (439.8706, 54.0971) (440.0521, 53.1847) (440.6588, 52.578) knots 0 0 0 0 1 1 1 1 projected
  spline S613 degree 3 poles (440.6588, 52.578) (441.2655, 51.9713) (442.1779, 51.7898) (442.9706, 52.1182) knots 0 0 0 0 1 1 1 1 projected
  spline S614 degree 3 poles (461.2088, 56.1993) (460.3508, 56.1993) (459.5773, 55.6825) (459.249, 54.8898) knots 0 0 0 0 1 1 1 1 projected
  spline S615 degree 3 poles (462.7088, 55.578) (462.311, 55.9758) (461.7714, 56.1993) (461.2088, 56.1993) knots 0 0 0 0 1 1 1 1 projected
  spline S616 degree 3 poles (459.249, 54.8898) (458.9206, 54.0971) (459.1021, 53.1847) (459.7088, 52.578) knots 0 0 0 0 1 1 1 1 projected
  spline S617 degree 3 poles (463.3301, 54.078) (463.3301, 54.6406) (463.1066, 55.1802) (462.7088, 55.578) knots 0 0 0 0 1 1 1 1 projected
  spline S618 degree 3 poles (459.7088, 52.578) (460.3155, 51.9713) (461.2279, 51.7898) (462.0206, 52.1182) knots 0 0 0 0 1 1 1 1 projected
  spline S619 degree 3 poles (462.0206, 52.1182) (462.8133, 52.4465) (463.3301, 53.22) (463.3301, 54.078) knots 0 0 0 0 1 1 1 1 projected
  spline S620 degree 3 poles (442.9706, 52.1182) (443.7633, 52.4465) (444.2801, 53.22) (444.2801, 54.078) knots 0 0 0 0 1 1 1 1 projected
  spline S621 degree 3 poles (443.6588, 17.478) (443.261, 17.8758) (442.7214, 18.0993) (442.1588, 18.0993) knots 0 0 0 0 1 1 1 1 projected
  spline S622 degree 3 poles (444.2801, 15.978) (444.2801, 16.5406) (444.0566, 17.0802) (443.6588, 17.478) knots 0 0 0 0 1 1 1 1 projected
  spline S623 degree 3 poles (442.9706, 14.0182) (443.7633, 14.3465) (444.2801, 15.12) (444.2801, 15.978) knots 0 0 0 0 1 1 1 1 projected
  spline S624 degree 3 poles (440.6588, 14.478) (441.2655, 13.8713) (442.1779, 13.6898) (442.9706, 14.0182) knots 0 0 0 0 1 1 1 1 projected
  spline S625 degree 3 poles (440.199, 16.7898) (439.8706, 15.9971) (440.0521, 15.0847) (440.6588, 14.478) knots 0 0 0 0 1 1 1 1 projected
  spline S626 degree 3 poles (442.1588, 18.0993) (441.3008, 18.0993) (440.5273, 17.5825) (440.199, 16.7898) knots 0 0 0 0 1 1 1 1 projected
  spline S627 degree 3 poles (443.6588, 36.528) (443.261, 36.9258) (442.7214, 37.1493) (442.1588, 37.1493) knots 0 0 0 0 1 1 1 1 projected
  spline S628 degree 3 poles (444.2801, 35.028) (444.2801, 35.5906) (444.0566, 36.1302) (443.6588, 36.528) knots 0 0 0 0 1 1 1 1 projected
  spline S629 degree 3 poles (442.1588, 37.1493) (441.3008, 37.1493) (440.5273, 36.6325) (440.199, 35.8398) knots 0 0 0 0 1 1 1 1 projected
  spline S630 degree 3 poles (440.199, 35.8398) (439.8706, 35.0471) (440.0521, 34.1347) (440.6588, 33.528) knots 0 0 0 0 1 1 1 1 projected
  spline S631 degree 3 poles (440.6588, 33.528) (441.2655, 32.9213) (442.1779, 32.7398) (442.9706, 33.0682) knots 0 0 0 0 1 1 1 1 projected
  spline S632 degree 3 poles (462.7088, 26.976) (462.311, 27.3738) (461.7714, 27.5973) (461.2088, 27.5973) knots 0 0 0 0 1 1 1 1 projected
  spline S633 degree 3 poles (461.2088, 27.5973) (460.0372, 27.5973) (459.0875, 26.6476) (459.0875, 25.476) knots 0 0 0 0 1 1 1 1 projected
  spline S634 degree 3 poles (463.3301, 25.476) (463.3301, 26.0386) (463.1066, 26.5782) (462.7088, 26.976) knots 0 0 0 0 1 1 1 1 projected
  spline S635 degree 3 poles (459.0875, 25.476) (459.0875, 24.3044) (460.0372, 23.3547) (461.2088, 23.3547) knots 0 0 0 0 1 1 1 1 projected
  spline S636 degree 3 poles (461.2088, 23.3547) (462.3804, 23.3547) (463.3301, 24.3044) (463.3301, 25.476) knots 0 0 0 0 1 1 1 1 projected
  spline S637 degree 3 poles (442.9706, 33.0682) (443.7633, 33.3965) (444.2801, 34.17) (444.2801, 35.028) knots 0 0 0 0 1 1 1 1 projected
  spline S638 degree 3 poles (339.4513, 34.9804) (339.4513, 35.543) (339.2278, 36.0826) (338.83, 36.4804) knots 0 0 0 0 1 1 1 1 projected
  spline S639 degree 3 poles (339.4513, 34.9804) (339.4513, 35.543) (339.2278, 36.0826) (338.83, 36.4804) knots 0 0 0 0 1 1 1 1 projected
  spline S640 degree 3 poles (339.4513, 34.9804) (339.4513, 35.543) (339.2278, 36.0826) (338.83, 36.4804) knots 0 0 0 0 1 1 1 1 projected
  spline S641 degree 3 poles (339.4513, 34.9804) (339.4513, 35.543) (339.2278, 36.0826) (338.83, 36.4804) knots 0 0 0 0 1 1 1 1 projected
  spline S642 degree 3 poles (339.4513, 34.9804) (339.4513, 35.543) (339.2278, 36.0826) (338.83, 36.4804) knots 0 0 0 0 1 1 1 1 projected
  spline S643 degree 3 poles (338.83, 36.4804) (338.4322, 36.8782) (337.8926, 37.1017) (337.33, 37.1017) knots 0 0 0 0 1 1 1 1 projected
  spline S644 degree 3 poles (338.83, 36.4804) (338.4322, 36.8782) (337.8926, 37.1017) (337.33, 37.1017) knots 0 0 0 0 1 1 1 1 projected
  spline S645 degree 3 poles (338.83, 36.4804) (338.4322, 36.8782) (337.8926, 37.1017) (337.33, 37.1017) knots 0 0 0 0 1 1 1 1 projected
  spline S646 degree 3 poles (338.83, 36.4804) (338.4322, 36.8782) (337.8926, 37.1017) (337.33, 37.1017) knots 0 0 0 0 1 1 1 1 projected
  spline S647 degree 3 poles (338.83, 36.4804) (338.4322, 36.8782) (337.8926, 37.1017) (337.33, 37.1017) knots 0 0 0 0 1 1 1 1 projected
  spline S648 degree 3 poles (337.33, 32.8591) (338.5016, 32.8591) (339.4513, 33.8088) (339.4513, 34.9804) knots 0 0 0 0 1 1 1 1 projected
  spline S649 degree 3 poles (337.33, 32.8591) (338.5016, 32.8591) (339.4513, 33.8088) (339.4513, 34.9804) knots 0 0 0 0 1 1 1 1 projected
  spline S650 degree 3 poles (337.33, 32.8591) (338.5016, 32.8591) (339.4513, 33.8088) (339.4513, 34.9804) knots 0 0 0 0 1 1 1 1 projected
  spline S651 degree 3 poles (337.33, 32.8591) (338.5016, 32.8591) (339.4513, 33.8088) (339.4513, 34.9804) knots 0 0 0 0 1 1 1 1 projected
  spline S652 degree 3 poles (337.33, 37.1017) (336.1584, 37.1017) (335.2087, 36.152) (335.2087, 34.9804) knots 0 0 0 0 1 1 1 1 projected
  spline S653 degree 3 poles (337.33, 37.1017) (336.1584, 37.1017) (335.2087, 36.152) (335.2087, 34.9804) knots 0 0 0 0 1 1 1 1 projected
  spline S654 degree 3 poles (337.33, 37.1017) (336.1584, 37.1017) (335.2087, 36.152) (335.2087, 34.9804) knots 0 0 0 0 1 1 1 1 projected
  spline S655 degree 3 poles (337.33, 37.1017) (336.1584, 37.1017) (335.2087, 36.152) (335.2087, 34.9804) knots 0 0 0 0 1 1 1 1 projected
  spline S656 degree 3 poles (337.33, 37.1017) (336.1584, 37.1017) (335.2087, 36.152) (335.2087, 34.9804) knots 0 0 0 0 1 1 1 1 projected
  spline S657 degree 3 poles (335.2087, 34.9804) (335.2087, 33.8088) (336.1584, 32.8591) (337.33, 32.8591) knots 0 0 0 0 1 1 1 1 projected
  spline S658 degree 3 poles (335.2087, 34.9804) (335.2087, 33.8088) (336.1584, 32.8591) (337.33, 32.8591) knots 0 0 0 0 1 1 1 1 projected
  spline S659 degree 3 poles (335.2087, 34.9804) (335.2087, 33.8088) (336.1584, 32.8591) (337.33, 32.8591) knots 0 0 0 0 1 1 1 1 projected
  spline S660 degree 3 poles (335.2087, 34.9804) (335.2087, 33.8088) (336.1584, 32.8591) (337.33, 32.8591) knots 0 0 0 0 1 1 1 1 projected
  spline S661 degree 3 poles (335.2087, 34.9804) (335.2087, 33.8088) (336.1584, 32.8591) (337.33, 32.8591) knots 0 0 0 0 1 1 1 1 projected
  spline S662 degree 3 poles (337.33, 32.8591) (338.5016, 32.8591) (339.4513, 33.8088) (339.4513, 34.9804) knots 0 0 0 0 1 1 1 1 projected
  point P0 (0, 0)
extrude "Extrusion1" add sketch "Sketch2" along normal blind 1.6
sketch "Sketch3" plane through (0, 0, 1.6) normal (0, 0, 1) x (1, 0, 0)
  line L0 (23.8588, 130.1384) -> (42.8588, 130.1384)
  line L1 (42.8588, 130.1384) -> (42.8588, 111.1384)
  line L2 (42.8588, 111.1384) -> (23.8588, 111.1384)
  line L3 (23.8588, 111.1384) -> (23.8588, 130.1384)
  arc A0 (35.4801, 120.6384) -> (33.3588, 122.7597) centre (33.3588, 120.6384) ccw projected
  line L4 (23.8588, 130.1384) -> (42.8588, 111.1384) construction
  line L5 (42.8588, 130.1384) -> (23.8588, 111.1384) construction
  line L6 (53.0988, 130.1384) -> (171.0988, 130.1384)
  line L7 (171.0988, 130.1384) -> (171.0988, 111.1384)
  line L8 (171.0988, 111.1384) -> (53.0988, 111.1384)
  line L9 (53.0988, 111.1384) -> (53.0988, 130.1384)
  line L10 (181.1148, 130.1384) -> (299.1148, 130.1384)
  line L11 (299.1148, 130.1384) -> (299.1148, 111.1384)
  line L12 (299.1148, 111.1384) -> (181.1148, 111.1384)
  line L13 (181.1148, 111.1384) -> (181.1148, 130.1384)
  line L14 (327.83, 101.5796) -> (384.93, 101.5796)
  line L15 (384.93, 101.5796) -> (384.93, 82.6444)
  line L16 (384.93, 82.6444) -> (327.83, 82.6444)
  line L17 (327.83, 82.6444) -> (327.83, 101.5796)
  line L18 (395.6338, 101.5796) -> (469.6338, 101.5796)
  line L19 (469.6338, 101.5796) -> (469.6338, 6.3796)
  line L20 (469.6338, 6.3796) -> (395.6338, 6.3796)
  line L21 (395.6338, 6.3796) -> (395.6338, 101.5796)
  line L22 (23.8588, 101.5796) -> (23.8588, 25.4296)
  line L23 (23.8588, 25.4296) -> (37.8588, 25.4296)
  line L24 (37.8588, 25.4296) -> (37.8588, 6.3796)
  line L25 (37.8588, 6.3796) -> (304.9568, 6.3796)
  line L26 (22.5, 6.25) -> (472.5, 6.25) projected
  line L27 (304.9568, 6.3796) -> (304.9568, 25.4296)
  line L28 (304.9568, 25.4296) -> (318.9568, 25.4296)
  line L29 (318.9568, 25.4296) -> (318.9568, 101.5796)
  line L30 (318.9568, 101.5796) -> (23.8588, 101.5796)
  line L31 (346.88, 63.5304) -> (346.88, 44.4804)
  line L32 (346.88, 44.4804) -> (327.83, 44.4804)
  line L33 (327.83, 44.4804) -> (327.83, 25.4804)
  line L34 (327.83, 25.4804) -> (384.93, 25.4804)
  line L35 (384.93, 25.4804) -> (384.93, 44.4804)
  line L36 (384.93, 44.4804) -> (365.88, 44.4804)
  line L37 (365.88, 44.4804) -> (365.88, 63.5304)
  line L38 (365.88, 63.5304) -> (346.88, 63.5304)
  arc A1 (40.1501, 92.0796) -> (38.0288, 94.2009) centre (38.0288, 92.0796) ccw construction
  circle A2 centre (38.0288, 92.0796) radius 2.5 construction
  arc A3 (311.5781, 92.0796) -> (309.4568, 94.2009) centre (309.4568, 92.0796) ccw construction
  circle A4 centre (309.4568, 92.0796) radius 2.5 construction
  arc A5 (358.5013, 54.0304) -> (356.38, 56.1517) centre (356.38, 54.0304) ccw construction
  circle A6 centre (356.38, 54.0304) radius 2.5 construction
  arc A7 (339.4513, 34.9804) -> (337.33, 37.1017) centre (337.33, 34.9804) ccw construction
  circle A8 centre (337.33, 34.9804) radius 2.5 construction
  arc A9 (377.5513, 34.9804) -> (375.43, 37.1017) centre (375.43, 34.9804) ccw construction
  circle A10 centre (375.43, 34.9804) radius 2.5 construction
  arc A11 (372.7753, 92.1444) -> (370.654, 94.2657) centre (370.654, 92.1444) ccw construction
  circle A12 centre (370.654, 92.1444) radius 2.5 construction
  arc A13 (344.1793, 92.1444) -> (342.058, 94.2657) centre (342.058, 92.1444) ccw construction
  circle A14 centre (342.058, 92.1444) radius 2.5 construction
  arc A15 (406.1801, 92.178) -> (404.0588, 94.2993) centre (404.0588, 92.178) ccw construction
  circle A16 centre (404.0588, 92.178) radius 2.5 construction
  arc A17 (463.3301, 92.178) -> (461.2088, 94.2993) centre (461.2088, 92.178) ccw construction
  circle A18 centre (461.2088, 92.178) radius 2.5 construction
  arc A19 (172.8941, 15.8796) -> (170.7728, 18.0009) centre (170.7728, 15.8796) ccw construction
  circle A20 centre (170.7728, 15.8796) radius 2.5 construction
  arc A21 (114.2201, 120.7084) -> (112.0988, 122.8297) centre (112.0988, 120.7084) ccw construction
  circle A22 centre (112.0988, 120.7084) radius 2.5 construction
  arc A23 (242.2361, 120.7364) -> (240.1148, 122.8577) centre (240.1148, 120.7364) ccw construction
  circle A24 centre (240.1148, 120.7364) radius 2.5 construction
  line L39 (432.6338, 92.178) -> (432.6338, 15.8796) construction
  line L40 (404.0588, 92.178) -> (432.6338, 92.178) construction
  line L41 (432.6338, 92.178) -> (461.2088, 92.178) construction
  arc A25 (42.5921, 34.9296) -> (40.4708, 37.0509) centre (40.4708, 34.9296) ccw construction
  circle A26 centre (40.4708, 34.9296) radius 2.5 construction
  point P0 (0, 0)
  dimension "d2" = 19
  dimension "d3" = 19
  dimension "d4" = 5
  dimension "d5" = 9.5
  dimension "d7" = 9.5
  dimension "d9" = 9.5
  dimension "d10" = 9.5
  dimension "d11" = 9.5
  dimension "d12" = 9.5
  dimension "d13" = 9.5
  dimension "d14" = 9.5
  dimension "d15" = 9.5
  dimension "d16" = 9.5
  dimension "d17" = 9.5
  dimension "d18" = 59
  dimension "d19" = 59
  dimension "d20" = 59
  dimension "d21" = 59
  dimension "d22" = 37
  dimension "d23" = 37
  dimension "d24" = 9.5
  dimension "d25" = 14
  dimension "d26" = 14
  constraints: 82 end point, 15 perpendicular, 13 centre point, 13 coincident, 12 equal radius, 11 parallel, 10 collinear, 7 horizontal, 6 point on line, 3 vertical, 2 midpoint
  measures "d2" distance of L0.start L0.end
  measures "d3" distance of L0.end L1.end
  measures "d4" diameter of A2
  measures "d5" distance from line of L30 A1.centre
  measures "d7" distance from line of L29 A4.centre
  measures "d9" distance from line of L16 A14.centre
  measures "d10" distance from line of L38 A6.centre
  measures "d11" distance from line of L34 A8.centre
  measures "d12" distance from line of L33 A7.centre
  measures "d13" distance from line of A6.centre L31
  measures "d14" distance from line of L37 A6.centre
  measures "d15" distance from line of L35 A10.centre
  measures "d16" distance from line of L36 A9.centre
  measures "d17" distance from line of L25 A20.centre
  measures "d18" distance from line of A21.centre L9
  measures "d19" distance from line of L7 A22.centre
  measures "d20" distance from line of L13 A24.centre
  measures "d21" distance from line of L11 A23.centre
  measures "d22" distance between parallel lines of L39 L21
  measures "d23" distance between parallel lines of L19 L39
  measures "d24" distance from line of L23 A26.centre
  measures "d25" distance between parallel lines of L24 L22
  measures "d26" distance between parallel lines of L27 L29
equation "\"d2\" = d3"
equation "\"d5\" = 0.5 * d3"
equation "\"d7\" = 0.5 * d3"
equation "\"d9\" = d5"
equation "\"d10\" = d5"
equation "\"d11\" = d5"
equation "\"d12\" = d5"
equation "\"d13\" = d5"
equation "\"d14\" = d5"
equation "\"d15\" = d5"
equation "\"d16\" = d5"
equation "\"d17\" = d5"
equation "\"d19\" = d18"
equation "\"d20\" = d18"
equation "\"d21\" = d18"
equation "\"d23\" = d22"
equation "\"d24\" = d5"
equation "\"d26\" = d25"
body "Solid1"
